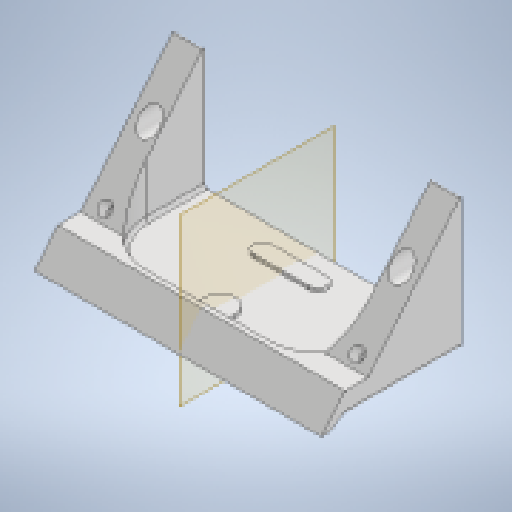
# Autodesk Inventor part: MS_podstawa
Saved by Autodesk Inventor 2023 (Build 270158000, 158)
## iProperties
Created: 2024-04-29
Part Number: MS_podstawa
Material: Ogólny
Document SubType Name: Modeling
Designer: kamil
Density: 1 g/cm^3
Appearance: Domyślna
Author: kamil
Autodesk Inventor part; units mm, degrees
ref_plane "YZ Plane" through (0, 0, 0) normal (1, 0, 0) x (0, 1, 0)
ref_plane "XZ Plane" through (0, 0, 0) normal (0, 1, 0) x (-1, 0, 0)
ref_plane "XY Plane" through (0, 0, 0) normal (0, 0, 1) x (1, 0, 0)
sketch "Szkic1" plane through (0, 0, 0) normal (0, 1, 0) x (-1, 0, 0)
  line L0 (9.0922, 8.517) -> (-72.9078, 8.517)
  line L1 (-72.9078, 8.517) -> (-72.9078, -31.483)
  line L2 (-72.9078, -31.483) -> (9.0922, -31.483)
  line L3 (9.0922, -31.483) -> (9.0922, 8.517)
  point P0 (0, 0)
  dimension "d0" = 82
  dimension "d1" = 40
  constraints: 8 end point, 2 parallel, 1 horizontal, 1 perpendicular
  measures "d0" distance of L2.end L1.end
  measures "d1" distance of L1.end L0.end
extrude "Wyciągnięcie proste1" add sketch "Szkic1" along normal blind 2
sketch "Szkic2" plane through (-9.0922, 0, -31.483) normal (-1, 0, 0) x (0, 0, 1)
  line L0 (40, 0) -> (40, 2) projected
  line L1 (0, 0) -> (40, 0) projected
  line L2 (0, 0) -> (40, 0) projected
  line L3 (40, 0) -> (40, 2) projected
  line L4 (0, 2) -> (40, 2) projected
  line L5 (0, 0) -> (0, 2) projected
  line L6 (40, -3) -> (35.8045, 2)
  line L7 (40, -3) -> (38, -3)
  line L8 (38, -3) -> (29.3397, 2)
  line L9 (40, 2) -> (0, 2) projected
  point P0 (31.483, 0)
  point P1 (40, 1)
  point P2 (37.4827, 0)
  point P3 (32.8038, 0)
  dimension "d4" = 3
  dimension "d5" = 50
  dimension "d6" = 2
  dimension "d11" = 150
  constraints: 6 end point, 2 point on line, 1 horizontal, 1 midpoint, 1 vertical alignment
  measures "d4" distance from line of L6.start L1
  measures "d5" angle of L4 L6
  measures "d6" distance of L6.start L7.end
  measures "d11" angle of L7 L8
extrude "Wyciągnięcie proste2" cut sketch "Szkic2" against normal through all contours L1 L6 L4 L0
extrude "Wyciągnięcie proste3" add sketch "Szkic2" against normal up to surface (82 mm away) contours L6 L7 L8 L1
sketch "Szkic4" plane through (-9.0922, 0, -31.483) normal (-1, 0, 0) x (0, 0, 1)
  line L0 (0, 0) -> (0, 2) projected
  line L1 (40, -3) -> (35.8045, 2) projected
  line L2 (40, -3) -> (35.8045, 2)
  line L3 (35.8045, 2) -> (0, 44.6701)
  line L4 (35.8045, 2) -> (0, 2) projected
  line L5 (0, 2) -> (0, 44.6701)
  point P0 (31.483, 0)
  constraints: 6 end point, 2 collinear, 1 vertical
extrude "Wyciągnięcie proste5" add sketch "Szkic4" against normal blind 10
sketch "Szkic5" plane through (-9.0922, 0, -31.483) normal (-1, 0, 0) x (0, 0, 1)
  line L0 (40, -3) -> (0, 44.6701) projected
  line L1 (36.1698, -6.2139) -> (-3.8302, 41.4562)
  line L2 (0, 2) -> (35.8045, 2) projected
  line L3 (0, 5) -> (34.9654, 5)
  line L4 (0, 44.6701) -> (0, 36.8915)
  line L5 (0, 0) -> (0, 44.6701) projected
  point P0 (31.483, 0)
  point P1 (26.7602, 5)
  point P2 (33.2872, 5)
  dimension "d17" = 5
  dimension "d18" = 3
  constraints: 6 end point, 2 parallel, 2 point on line
  measures "d17" distance between parallel lines of L0 L1
  measures "d18" distance between parallel lines of L2 L3
extrude "Wyciągnięcie proste6" cut sketch "Szkic5" against normal through all contours L3 L1 L4 L0
sketch "Szkic6" plane through (72.9078, 0, -31.483) normal (0, 0, -1) x (-1, 0, 0)
  circle A0 centre (77, 22.5) radius 2 projected
  circle A1 centre (77, 22.5) radius 1.6
  circle A2 centre (77, 22.5) radius 3
  point P0 (72.9078, 0)
  dimension "d21" = 3.2
  dimension "d22" = 6
  constraints: 2 centre point, 2 coincident
  measures "d21" diameter of A1
  measures "d22" diameter of A2
extrude "Wyciągnięcie proste7" cut sketch "Szkic6" against normal through all contours A0 | A1 | A2
sketch "Szkic7" plane through (72.9078, 0, -31.483) normal (0, 0, -1) x (-1, 0, 0)
  circle A0 centre (77, 22.5) radius 3 projected
  circle A1 centre (77, 22.5) radius 1.6
  point P0 (72.9078, 0)
  dimension "d25" = 3.2
  constraints: 1 centre point, 1 coincident
  measures "d25" diameter of A1
extrude "Wyciągnięcie proste8" add sketch "Szkic7" against normal blind 5
sketch "Szkic8" plane through (-9.0922, 36.8915, -31.483) normal (0, 0.6427876, 0.7660444) x (1, 0, 0)
  ellipse E0 centre (5, -18.7868) end of major axis (5, -22.703) minor radius 3 projected
  line L0 (10, 0) -> (10, -41.6314) projected
  line L1 (0, 0) -> (10, 0) projected
  line L2 (0, -41.6314) -> (0, 0) projected
  line L3 (0, -41.6314) -> (10, -41.6314) projected
  ellipse E1 centre (5, -18.7868) end of major axis (5, -22.703) minor radius 3 construction
  point P0 (9.0922, -48.4974)
  point P1 (5, -38.6314)
  dimension "d28" = 3
  constraints: 1 vertical alignment, 2 other
  measures "d28" distance from line of L3 point (5, -38.631)
hole "Otwór1" at (-4.0922, 7.2981, -6.6512) direction (0, -0.6427876, -0.7660444) diameter 3.2 depth 8 counterbore diameter 4 counterbore depth 4
sketch "Szkic9" plane through (-9.0922, 0, -31.483) normal (-1, 0, 0) x (0, 0, 1)
  line L0 (26.7602, 5) -> (0, 36.8915) projected
  line L1 (0, 2) -> (35.8045, 2) projected
  line L2 (40, -3) -> (33.2872, 5) projected
  line L3 (33.2872, 5) -> (26.7602, 5) projected
  line L4 (0, 36.8915) -> (26.7602, 5) projected
  line L5 (26.7602, 5) -> (26.7602, 2)
  point P0 (31.483, 0)
  constraints: 2 end point, 1 perpendicular, 1 point on line
extrude "Wyciągnięcie proste9" add sketch "Szkic9" against normal up to surface (82 mm away)
ref_plane "Płaszczyzna konstrukcyjna1" through (31.9078, 0, -31.483) normal (1, 0, 0) x (0, 0, -1)
mirror "Odbij1" about plane through (31.9078, 0, -31.483) normal (1, 0, 0) of "Otwór1", "Wyciągnięcie proste8", "Wyciągnięcie proste7", "Wyciągnięcie proste6", "Wyciągnięcie proste5"
sketch "Szkic10" plane through (0.9078, 2, -4.7228) normal (0, 0, -1) x (-1, 0, 0)
  line L0 (-62, 3) -> (-62, 0) projected
  line L1 (0, 0) -> (-62, 0) projected
  line L2 (0, 3) -> (0, 0) projected
  line L3 (0, 3) -> (-62, 3) projected
  point P0 (0.9078, -2)
extrude "Wyciągnięcie proste10" cut sketch "Szkic10" against normal blind 3.5
sketch "Szkic13" plane through (0.9078, 0, -31.483) normal (1, 0, 0) x (0, 0, -1)
  line L0 (0, 2) -> (-30.2602, 2) projected
  line L1 (0, 2) -> (0, 36.8915) projected
  line L2 (0, 36.8915) -> (-26.7602, 5) projected
  line L3 (-30.2602, 5) -> (-26.7602, 5) projected
  line L4 (-30.2602, 5) -> (-30.2602, 2) projected
  point P0 (-31.483, 0)
extrude "Wyciągnięcie proste12" cut sketch "Szkic13" against normal blind 1.5
mirror "Odbij2" about plane through (31.9078, 0, -31.483) normal (1, 0, 0) of "Wyciągnięcie proste12"
sketch "Szkic14" plane through (0, 2, 0) normal (0, 1, 0) x (1, 0, 0)
  line L0 (-0.5922, 1.2228) -> (-0.5922, 4.7228) projected
  line L1 (64.4078, 4.7228) -> (64.4078, 1.2228) projected
  line L2 (48.9078, 0.183) -> (14.9078, 0.183)
  line L3 (-0.5922, 1.2228) -> (64.4078, 1.2228) projected
  line L4 (64.4078, 1.2228) -> (-0.5922, 1.2228)
  line L5 (-0.5922, 1.2228) -> (-0.5922, -0.2772)
  line L6 (-0.5922, -0.2772) -> (64.4078, -0.2772)
  line L7 (64.4078, -0.2772) -> (64.4078, 1.2228)
  point P0 (0, 0)
  dimension "d44" = 1.5
  constraints: 10 end point, 2 horizontal, 2 parallel, 1 perpendicular, 2 other
  measures "d44" distance of L5.end L4.end
extrude "Wyciągnięcie proste13" cut sketch "Szkic14" along normal through all
fillet "Zaokrąglenie1" radius 15 2 edges at (-0.5922, 3.5, 0.2772) (64.4078, 3.5, 0.2772)
sketch "Szkic15" plane through (0, 2, 0) normal (0, 1, 0) x (1, 0, 0)
  circle A0 centre (32.0078, 3.483) radius 1.6
  line L0 (49.4078, -0.2772) -> (14.4078, -0.2772) projected
  circle A1 centre (32.0078, 3.483) radius 4.2613
  line L1 (36.2692, 3.483) -> (36.2692, -0.2772)
  line L2 (14.4078, -0.2772) -> (49.4078, -0.2772) projected
  line L3 (27.7465, 3.483) -> (27.7465, -0.2772)
  line L4 (24.0078, 23.483) -> (40.0078, 23.483) construction
  line L5 (24.0078, 20.983) -> (40.0078, 20.983)
  line L6 (40.0078, 25.983) -> (24.0078, 25.983)
  arc A2 (24.0078, 25.983) -> (24.0078, 20.983) centre (24.0078, 23.483) ccw
  arc A3 (40.0078, 20.983) -> (40.0078, 25.983) centre (40.0078, 23.483) ccw
  point P0 (0, 0)
  point P1 (32.0078, 23.483)
  point P2 (27.7465, -0.2772)
  point P3 (36.2692, -0.2772)
  dimension "d48" = 8
  dimension "d49" = 5
  dimension "d50" = 20
  constraints: 12 end point, 6 point on circle, 5 tangent, 4 centre point, 2 point on line, 1 coincident, 1 horizontal, 1 midpoint, 1 parallel, 1 perpendicular, 1 vertical, 1 vertical alignment, 2 other
  measures "d48" distance of point (32.008, 23.483) L4.end
  measures "d49" diameter of A3
  measures "d50" distance of point (32.008, 23.483) A0.centre
ref_plane "Płaszczyzna konstrukcyjna2" through (14.9078, 3, -31.483) normal (0, -1, 0) x (1, 0, 0)
extrude "Wyciągnięcie proste14" add sketch "Szkic15" along normal up to surface (1 mm away) contours A0 | L0 A1 L1 | L0 A1 | L0 L3 A1 | A2 L6 A3 L5 picked at (32.0721, 0.4468)
fillet "Zaokrąglenie2" radius 1 6 edges at (64.4078, 2, -23.1029) (42.8385, 2, 0.2772) (60.0144, 2, -4.1162) (21.0772, 2, 0.2772) (-0.5922, 2, -23.1029) (3.8012, 2, -4.1162)
sketch "Szkic16" plane through (-9.0922, 0, -31.483) normal (-1, 0, 0) x (0, 0, 1)
  line L0 (40, -3) -> (33.2872, 5) projected
  line L1 (33.2872, 5) -> (26.7602, 5) projected
  line L2 (26.7602, 5) -> (0, 36.8915) projected
  line L3 (0, 0) -> (0, 36.8915) projected
  line L4 (0, 0) -> (32.8038, 0) projected
  line L5 (32.8038, 0) -> (38, -3) projected
  line L6 (38, -3) -> (40, -3) projected
  line L7 (32.8038, 0) -> (38, -3) projected
  line L8 (34.5359, -1) -> (0, -1)
  line L9 (0, -1) -> (0, 0)
  point P0 (31.483, 0)
  dimension "d54" = 1
  constraints: 4 end point, 1 horizontal, 1 point on line, 1 vertical
  measures "d54" distance between parallel lines of L8 L4
extrude "Wyciągnięcie proste15" add sketch "Szkic16" against normal up to surface (82 mm away) contours L8 L9 L4 L5
fillet "Zaokrąglenie3" radius 0.3 2 edges at (68.6578, 36.8915, -31.483) (-4.8422, 36.8915, -31.483)
fillet "Zaokrąglenie4" radius 1 2 edges at (-9.0922, -1, -14.2151) (72.9078, -1, -14.2151)
fillet "Zaokrąglenie5" radius 1 4 edges at (-9.0922, -0.5, 2.1869) (-9.0922, -2, 4.7849) (72.9078, -0.5, 2.1869) (72.9078, -2, 4.7849)
fillet "Zaokrąglenie6" radius 2 6 edges at (71.9079, -1, 3.0529) (72.6211, -0.7009, 3.1329) (-8.0923, -1, 3.0529) (-8.8055, -0.7009, 3.1329) (-8.0922, -1, 3.0529) (31.9078, -1, 3.0529)
sketch "Szkic18" plane through (32.0078, 3, -3.483) normal (0, 1, 0) x (1, 0, 0)
  circle A0 centre (0, 0) radius 1.6
  point P0 (-32.0078, -3.483)
  constraints: 1 centre point, 2 other
hole "Otwór2" at (32.0078, 3, -3.483) direction (0, -1, 0) diameter 3.2 depth 9 counterbore diameter 4.1 counterbore depth 3.5
sketch "Szkic19" plane through (-8.0922, -1, -31.483) normal (0, -1, 0) x (1, 0, 0)
  circle A0 centre (40.1, 28) radius 1.6 projected
  line L0 (0, 34) -> (80, 34) projected
  line L1 (0, 0) -> (0, 34) projected
  line L2 (0, 0) -> (80, 0) projected
  line L3 (80, 34) -> (80, 0) projected
  line L4 (1, 33) -> (79, 33)
  line L5 (79, 33) -> (79, 1)
  line L6 (79, 1) -> (1, 1)
  line L7 (1, 1) -> (1, 33)
  line L8 (81, 33.2872) -> (-1, 33.2872) projected
  line L9 (40, 33.2872) -> (40, 1)
  line L10 (11, 33) -> (11, 22)
  line L11 (11, 22) -> (40, 22)
  line L12 (1, 12) -> (40, 12)
  arc A1 (35.8387, 28) -> (44.3613, 28) centre (40.1, 28) ccw projected
  line L13 (69, 33) -> (69, 22)
  line L14 (69, 22) -> (40, 22)
  line L15 (79, 12) -> (40, 12)
  point P0 (8.0922, 31.483)
  dimension "d68" = 1
  dimension "d69" = 10
  dimension "d70" = 10
  dimension "d71" = 11
  constraints: 22 end point, 4 point on line, 3 symmetric about line, 2 midpoint, 1 horizontal, 1 perpendicular, 1 vertical, 3 other
  measures "d68" distance between parallel lines of L1 L7
  measures "d69" distance between parallel lines of L10 L7
  measures "d70" distance between parallel lines of L12 L11
  measures "d71" distance of L10.start L10.end
extrude "Wyciągnięcie proste16" cut sketch "Szkic19" against normal blind 1.5 contours L10 L11 L9 L12 L7 L4 | L4 L5 L15 L9 L14 L13
fillet "Zaokrąglenie7" radius 1 8 edges at (2.9078, -0.25, 1.517) (-7.0922, -0.25, 1.517) (2.9078, -0.25, -9.483) (-7.0922, -0.25, -19.483) (60.9078, -0.25, -9.483) (60.9078, -0.25, 1.517) (70.9078, -0.25, 1.517) (70.9078, -0.25, -19.483)
sketch "Szkic20" plane through (-8.0922, 0.5, -31.483) normal (0, -1, 0) x (1, 0, 0)
  arc A0 (78, 12) -> (79, 13) centre (78, 13) ccw projected
  line L0 (79, 32) -> (79, 13) projected
  arc A1 (79, 32) -> (78, 33) centre (78, 32) ccw projected
  line L1 (70, 33) -> (78, 33) projected
  arc A2 (70, 33) -> (69, 32) centre (70, 32) ccw projected
  line L2 (69, 23) -> (69, 32) projected
  arc A3 (68, 22) -> (69, 23) centre (68, 23) ccw projected
  line L3 (12, 22) -> (68, 22) projected
  arc A4 (11, 23) -> (12, 22) centre (12, 23) ccw projected
  line L4 (11, 32) -> (11, 23) projected
  arc A5 (11, 32) -> (10, 33) centre (10, 32) ccw projected
  line L5 (2, 33) -> (10, 33) projected
  arc A6 (2, 33) -> (1, 32) centre (2, 32) ccw projected
  line L6 (1, 13) -> (1, 32) projected
  arc A7 (1, 13) -> (2, 12) centre (2, 13) ccw projected
  line L7 (78, 12) -> (2, 12) projected
  circle A8 centre (75.5, 15.5) radius 3.5
  circle A9 centre (4.5, 15.5) radius 3.5
  line L8 (78, 12) -> (2, 12) projected
  line L9 (79, 32) -> (79, 13) projected
  line L10 (1, 13) -> (1, 32) projected
  point P0 (8.0922, 31.483)
  dimension "d75" = 7
  dimension "d76" = 7
  constraints: 4 tangent, 2 centre point
  measures "d75" diameter of A8
  measures "d76" diameter of A9
hole "Otwór3" at (-3.5922, 0.5, -15.983) at (67.4078, 0.5, -15.983) direction (0, 1, 0) diameter 2 depth 6
sketch "Szkic21" plane through (-8.0922, -1, -31.483) normal (0, -1, 0) x (1, 0, 0)
  line L0 (57, 0) -> (57, 31.3)
  line L1 (71.5, 0) -> (71.5, 16.7602) projected
  line L2 (78, 12) -> (2, 12) projected
  line L3 (69.5, 2) -> (59, 2)
  line L4 (59, 2) -> (59, 12)
  line L5 (59, 12) -> (69.5, 12)
  line L6 (69.5, 12) -> (69.5, 2)
  point P0 (8.0922, 31.483)
  point P1 (69.5, 12)
  point P2 (59, 12)
  dimension "d84" = 2
  dimension "d85" = 2
  dimension "d86" = 0
  dimension "d87" = 10
  constraints: 10 end point, 2 parallel, 1 horizontal, 1 perpendicular, 1 vertical, 2 other
  measures "d84" distance between parallel lines of L0 L4
  measures "d85" distance between parallel lines of L6 L1
  measures "d86" distance between parallel lines of L2 L5
  measures "d87" distance between parallel lines of L3 L5
extrude "Wyciągnięcie proste17" cut sketch "Szkic21" against normal up to surface (1.5 mm away)
sketch "Szkic22" plane through (-8.0922, 0.5, -31.483) normal (0, -1, 0) x (1, 0, 0)
  line L0 (69.5, 12) -> (69.5, 2) projected
  line L1 (69.5, 2) -> (59, 2) projected
  line L2 (59, 2) -> (59, 12) projected
  line L3 (69.5, 2) -> (69.5, 12) projected
  line L4 (69.5, 6) -> (59, 6)
  point P0 (8.0922, 31.483)
  dimension "d90" = 4
  constraints: 2 end point, 2 point on line, 1 perpendicular
  measures "d90" distance between parallel lines of L1 L4
extrude "Wyciągnięcie proste18" cut sketch "Szkic22" against normal up to surface (1.5 mm away)
fillet "Zaokrąglenie8" radius 1 4 edges at (61.4078, -0.25, -19.483) (50.9078, -0.25, -19.483) (61.4078, 0.5, -29.483) (50.9078, 0.5, -29.483)
fillet "Zaokrąglenie9" radius 1 2 edges at (50.9078, 1.25, -25.483) (61.4078, 1.25, -25.483)
sketch "Szkic23" plane through (-9.0922, 5, -4.7228) normal (-1, 0, 0) x (0, 0, 1)
  line L0 (-13.5902, 10.1) -> (-9.1902, 10.1)
  line L1 (-9.1902, 10.1) -> (-9.1902, 7.7)
  line L2 (-13.5902, 7.7) -> (-13.5902, 10.1)
  line L3 (-9.1902, 7.7) -> (-13.5902, 7.7)
  line L4 (-15.5902, 5.7) -> (-15.5902, 12.1)
  line L5 (-15.5902, 12.1) -> (-7.1902, 12.1)
  line L6 (-7.1902, 12.1) -> (-7.1902, 5.7)
  line L7 (-7.1902, 5.7) -> (-15.5902, 5.7)
  point P0 (4.7228, -5)
  dimension "d95" = 2
  constraints: 16 end point, 2 horizontal, 2 vertical, 7 other
  measures "d95" distance between parallel lines of L3 L7
extrude "Wyciągnięcie proste19" cut sketch "Szkic23" against normal blind 10 contours L0 L1 L3 L2 | L4 L5 L6 L7
fillet "Zaokrąglenie10" radius 0.2 2 edges at (-4.7094, 13.5689, -11.913) (-4.8422, 17.1, -14.8759)
fillet "Zaokrąglenie11" radius 0.5 3 edges at (-4.8422, 10.7, -20.313) (-4.7094, 10.7, -11.913) (-4.8422, 17.1, -20.313)
sketch "Szkic24" plane through (72.9078, 5, 1.8042) normal (1, 0, 0) x (0, 0, -1)
  line L0 (24.4372, 7.7) -> (24.4372, 10.1)
  line L1 (20.0372, 7.7) -> (24.4372, 7.7)
  line L2 (20.0372, 10.1) -> (20.0372, 7.7)
  line L3 (24.4372, 10.1) -> (20.0372, 10.1)
  line L4 (26.4372, 5.7) -> (26.4372, 12.1)
  line L5 (26.4372, 12.1) -> (18.0372, 12.1)
  line L6 (18.0372, 12.1) -> (18.0372, 5.7)
  line L7 (18.0372, 5.7) -> (26.4372, 5.7)
  point P0 (1.8042, -5)
  dimension "d100" = 2
  constraints: 16 end point, 2 horizontal, 2 vertical, 7 other
  measures "d100" distance between parallel lines of L1 L7
extrude "Wyciągnięcie proste20" cut sketch "Szkic24" against normal blind 10 contours L1 L2 L3 L0 | L7 L6 L5 L4
fillet "Zaokrąglenie12" radius 0.5 4 edges at (68.6578, 10.7, -16.233) (68.6578, 17.1, -16.233) (68.6578, 17.1, -24.633) (68.6578, 10.7, -24.633)
